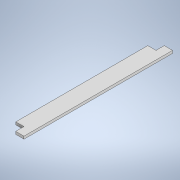
# Autodesk Inventor part: Top Sheet Metal Left
Saved by Autodesk Inventor 2020 (Build 240168000, 168)
## iProperties
Created: 2020-03-19
Part Number: Top Sheet Metal Left
Material: Generic
Document SubType Name: Modeling
Designer: Peter
Density: 1 g/cm^3
Appearance: Default
Author: Peter
Autodesk Inventor part; units mm, degrees
ref_plane "YZ Plane" through (0, 0, 0) normal (1, 0, 0) x (0, 1, 0)
ref_plane "XZ Plane" through (0, 0, 0) normal (0, 1, 0) x (-1, 0, 0)
ref_plane "XY Plane" through (0, 0, 0) normal (0, 0, 1) x (1, 0, 0)
sketch "Sketch1" plane through (0, 0, 0) normal (0, 1, 0) x (-1, 0, 0)
  line L0 (0, 0) -> (-40, 0)
  line L1 (-40, 0) -> (-40, -360)
  line L2 (-40, -360) -> (0, -360)
  line L3 (0, -360) -> (0, 0)
  line L4 (0, 0) -> (-20, 0)
  line L5 (-20, 0) -> (-20, -20)
  line L6 (-20, -20) -> (0, -20)
  line L7 (0, -20) -> (0, 0)
  line L8 (0, -360) -> (-20, -360)
  line L9 (-20, -360) -> (-20, -340)
  line L10 (-20, -340) -> (0, -340)
  line L11 (0, -340) -> (0, -360)
  point P0 (0, -20)
  dimension "d0" = 360
  dimension "d1" = 20
  dimension "d2" = 20
  dimension "d3" = 20
  dimension "d4" = 20
  dimension "d5" = 40
  constraints: 24 end point, 6 parallel, 3 horizontal, 3 perpendicular
  measures "d0" distance of L0.end L1.end
  measures "d1" distance of L6.end L5.end
  measures "d2" distance of L4.end L5.end
  measures "d3" distance of L9.end L10.end
  measures "d4" distance of L8.end L9.end
  measures "d5" distance between parallel lines of L1 L3
extrude "Extrusion1" add sketch "Sketch1" along normal blind 6.35 contours L5 L6 L3 L10 L9 L2 L1 L0
equation "\"d0\" = base_y_dim - 2 * extrusion_dim"
equation "\"d1\" = extrusion_dim"
equation "\"d2\" = extrusion_dim"
equation "\"d3\" = extrusion_dim"
equation "\"d4\" = extrusion_dim"
equation "\"d5\" = ceiling_width"
equation "\"d6\" = top_sheet_thickness"
equation "\"base_thickness\" = 12.7"
equation "\"extrusion_dim\" = 20"
equation "\"top_sheet_thickness\" = 6.35"
equation "\"ceiling_width\" = 40"
equation "\"base_y_dim\" = 400"
body "Solid1"
